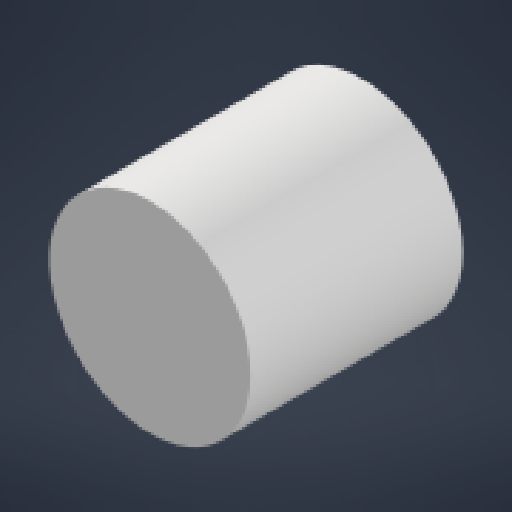
# Autodesk Inventor part: FalseAxle
Saved by Autodesk Inventor 2023 (Build 270158000, 158)
## iProperties
Created: 2023-08-11
Part Number: FalseAxle
Material: Generic
Document SubType Name: Modeling
Designer: Izack Waczko
Density: 1 g/cm^3
Appearance: Default
Author: Izack Waczko
Autodesk Inventor part; units mm, degrees
ref_plane "YZ Plane" through (0, 0, 0) normal (1, 0, 0) x (0, 1, 0)
ref_plane "XZ Plane" through (0, 0, 0) normal (0, 1, 0) x (-1, 0, 0)
ref_plane "XY Plane" through (0, 0, 0) normal (0, 0, 1) x (1, 0, 0)
sketch "Sketch1" plane through (0, 0, 0) normal (0, 0, 1) x (1, 0, 0)
  line L0 (3.4024, -4.5) -> (3.4024, 4.5) projected
  line L1 (-44.3976, 4.5) -> (-44.3976, -4.5) projected
  line L2 (3.4024, 0) -> (-44.3976, 0) construction
  circle A0 centre (-20.4976, 0) radius 28.5
  point P0 (0, 0)
  dimension "d0" = 57
  constraints: 3 midpoint, 2 end point, 1 centre point
  measures "d0" diameter of A0
extrude "Extrusion1" add sketch "Sketch1" along normal mid plane 60
body "Solid1"
